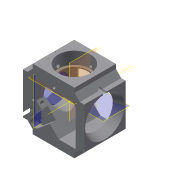
# Autodesk Inventor part: 20_Cube_Insert_Filter_25mm
Saved by Autodesk Inventor 2022 (Build 260153000, 153)
## iProperties
Created: 2019-07-01
Part Number: 20_Cube_Insert_Filter_25mm
Material: Generic
Document SubType Name: Modeling
Designer: diederichbenedict
Density: 1 g/cm^3
Appearance: Default
Author: diederichbenedict
Autodesk Inventor part; units mm, degrees
ref_plane "YZ Plane" through (0, 0, 0) normal (1, 0, 0) x (0, 1, 0)
ref_plane "Work Plane1" through (0, 0, 10) normal (0, 0, 1) x (1, 0, 0)
sketch "Sketch1" plane through (0, 0, 10) normal (0, 0, 1) x (1, 0, 0)
  line L0 (-4.029928, -0.353838) -> (-2.232156, 1.443934) construction
  arc A0 (-1.443934, 2.232156) -> (-2.232156, 1.443934) centre (-0.929928, 0.929928) ccw construction
  line L1 (-1.443934, 2.232156) -> (0.353838, 4.029928) construction
  line L2 (-37.829928, 42.829928) -> (-37.829928, 37.829928) construction
  line L3 (-37.829928, 37.829928) -> (-42.920801, 37.829928) construction
  line L4 (-37.829928, 42.213694) -> (-37.829928, 45.829928) construction
  line L5 (-37.829928, 45.829928) -> (-4.029928, 45.829928) construction
  line L6 (-4.029928, 45.829928) -> (-4.029928, 42.213694) construction
  line L7 (-4.029928, 4.029928) -> (0.353838, 4.029928)
  circle A1 centre (-20.929928, 20.929928) radius 17.5
  line L8 (-20.929928, 58.972273) -> (17.112417, 20.929928) construction
  line L9 (17.112417, 20.929928) -> (-20.929928, -17.112417) construction
  line L10 (-20.929928, -17.112417) -> (-58.972273, 20.929928) construction
  line L11 (-58.972273, 20.929928) -> (-20.929928, 58.972273) construction
  line L12 (-20.929928, 58.972273) -> (-20.929928, -17.112417) construction
  line L13 (17.112417, 20.929928) -> (-58.972273, 20.929928) construction
  line L14 (-20.929928, 58.972273) -> (32.870072, 58.972273) construction
  line L15 (-43.429928, 43.429928) -> (1.570072, 43.429928) construction
  line L16 (1.570072, 43.429928) -> (1.570072, -1.570072) construction
  line L17 (1.570072, -1.570072) -> (-43.429928, -1.570072) construction
  line L18 (-43.429928, -1.570072) -> (-43.429928, 43.429928) construction
  line L19 (-43.429928, 43.429928) -> (1.570072, -1.570072) construction
  line L20 (1.570072, 43.429928) -> (-43.429928, -1.570072) construction
  line L21 (-43.429928, 5.387583) -> (-43.429928, 36.472273)
  line L22 (-43.429928, 36.472273) -> (-36.472273, 43.429928)
  line L23 (-36.472273, 43.429928) -> (-5.387583, 43.429928)
  line L24 (-5.387583, 43.429928) -> (1.570072, 36.472273)
  line L25 (1.570072, 36.472273) -> (1.570072, 5.387583)
  line L26 (1.570072, 5.387583) -> (-5.387583, -1.570072)
  line L27 (-5.387583, -1.570072) -> (-36.472273, -1.570072)
  line L28 (-36.472273, -1.570072) -> (-43.429928, 5.387583)
  line L29 (-4.029928, 42.213694) -> (-37.829928, 42.213694)
  line L30 (-4.029928, -0.353838) -> (-4.029928, 4.029928)
  circle A2 centre (-20.929928, 20.929928) radius 1.5
  line L31 (-10.929928, 10.929928) -> (-30.929928, 10.929928) construction
  line L32 (-30.929928, 10.929928) -> (-30.929928, 30.929928) construction
  line L33 (-30.929928, 30.929928) -> (-10.929928, 30.929928) construction
  line L34 (-10.929928, 30.929928) -> (-10.929928, 10.929928) construction
  line L35 (-10.929928, 10.929928) -> (-30.929928, 30.929928) construction
  line L36 (-30.929928, 10.929928) -> (-10.929928, 30.929928) construction
  circle A3 centre (-30.929928, 30.929928) radius 1.4
  circle A4 centre (-30.929928, 10.929928) radius 1.4
  circle A5 centre (-10.929928, 10.929928) radius 1.4
  line L37 (-45.829928, 37.829928) -> (-42.072273, 37.829928) construction
  line L38 (-42.172273, 37.729928) -> (-45.829928, 37.729928)
  line L39 (-45.829928, 37.729928) -> (-45.829928, 4.129928)
  line L40 (-45.829928, 4.129928) -> (-42.172273, 4.129928)
  line L41 (-42.172273, 4.129928) -> (-42.172273, 37.729928)
  line L42 (-45.829928, 4.029928) -> (-42.072273, 4.029928) construction
  line L43 (-45.829928, 37.829928) -> (-42.072273, 37.829928)
  line L44 (-37.729928, 45.829928) -> (-4.129928, 45.829928)
  line L45 (-4.129928, 45.829928) -> (-4.129928, 42.172273)
  line L46 (-4.129928, 42.172273) -> (-37.729928, 42.172273)
  line L47 (-37.729928, 42.172273) -> (-37.729928, 45.829928)
  line L48 (0.470072, 37.829928) -> (0.470072, 4.029928) construction
  line L49 (0.470072, 4.029928) -> (3.970072, 4.029928) construction
  line L50 (3.970072, 37.829928) -> (3.970072, 4.029928) construction
  line L51 (0.470072, 37.829928) -> (3.970072, 37.829928) construction
  line L52 (-45.829928, -3.970072) -> (-4.029928, -3.970072) construction
  line L53 (0.312417, 37.729928) -> (3.970072, 37.729928)
  line L54 (3.970072, 37.729928) -> (3.970072, 4.129928)
  line L55 (3.970072, 4.129928) -> (0.312417, 4.129928)
  line L56 (0.312417, 4.129928) -> (0.312417, 37.729928)
  line L57 (-4.171349, -0.353838) -> (-37.729928, -0.353838)
  line L58 (-37.729928, -0.353838) -> (-37.729928, -3.970072)
  line L59 (-37.729928, -3.970072) -> (-4.171349, -3.970072)
  line L60 (-4.171349, -3.970072) -> (-4.171349, -0.353838)
  point P0 (-37.829928, 4.029928)
  dimension "d18" = 53.8
  dimension "d19" = 45
  dimension "d20" = 53.8
  dimension "d21" = 45
  dimension "d22" = 45
  dimension "d30" = 20
  dimension "d31" = 20
  dimension "d32" = 2.8
  dimension "d33" = 2.8
  dimension "d34" = 2.8
  dimension "d35" = 3
  dimension "d36" = 0.1
  dimension "d37" = 0.1
  dimension "d38" = 0.1
  dimension "d39" = 0.1
  constraints: 86 end point, 21 point on line, 14 parallel, 8 perpendicular, 7 horizontal, 7 midpoint, 4 centre point, 4 coincident, 1 equal length
  measures "d18" distance of L8.start L8.end
  measures "d19" angle of L8 L14
  measures "d20" distance of L8.end L9.end
  measures "d21" distance of L16.end L17.end
  measures "d22" distance of L15.end L16.end
  measures "d30" distance of L32.end L33.end
  measures "d31" distance of L31.end L32.end
  measures "d32" diameter of A3
  measures "d33" diameter of A4
  measures "d34" diameter of A5
  measures "d35" diameter of A2
  measures "d36" distance between parallel lines of L38 L43
  measures "d37" distance between parallel lines of L40 L42
  measures "d38" distance between parallel lines of L45 L6
  measures "d39" distance between parallel lines of L4 L47
sketch "Sketch1 outline for Extrusion1" plane through (0, 0, 10) normal (0, 0, 1) x (1, 0, 0)
  line L0 (-37.729928, -3.970072) -> (-4.171349, -3.970072)
  line L1 (-4.171349, -3.970072) -> (-4.171349, -0.353838)
  line L2 (0.312417, 4.129928) -> (-4.171349, -0.353838)
  line L3 (0.312417, 4.129928) -> (3.970072, 4.129928)
  line L4 (3.970072, 4.129928) -> (3.970072, 37.729928)
  line L5 (3.970072, 37.729928) -> (0.312417, 37.729928)
  line L6 (-4.129928, 42.172273) -> (0.312417, 37.729928)
  line L7 (-4.129928, 42.172273) -> (-4.129928, 45.829928)
  line L8 (-4.129928, 45.829928) -> (-37.729928, 45.829928)
  line L9 (-37.729928, 45.829928) -> (-37.729928, 42.172273)
  line L10 (-42.172273, 37.729928) -> (-37.729928, 42.172273)
  line L11 (-42.172273, 37.729928) -> (-45.829928, 37.729928)
  line L12 (-45.829928, 37.729928) -> (-45.829928, 4.129928)
  line L13 (-45.829928, 4.129928) -> (-42.172273, 4.129928)
  line L14 (-37.688507, -0.353838) -> (-42.172273, 4.129928)
  line L15 (-37.688507, -0.353838) -> (-37.729928, -0.353838)
  line L16 (-37.729928, -0.353838) -> (-37.729928, -3.970072)
extrude "Extrusion1" add sketch "Sketch1 outline for Extrusion1" along normal blind 33.8
sketch "Skizze4" plane through (0, 0, 43.8) normal (0, 0, 1) x (1, 0, 0)
  line L0 (-37.729928, 42.172273) -> (-42.172273, 37.729928)
  line L1 (-42.172273, 37.729928) -> (-45.829928, 37.729928)
  line L2 (-45.829928, 37.729928) -> (-45.829928, 4.129928) construction
  line L3 (-45.829928, 4.129928) -> (-42.172273, 4.129928)
  line L4 (-42.172273, 4.129928) -> (-37.688507, -0.353838)
  line L5 (-37.688507, -0.353838) -> (-37.729928, -0.353838)
  line L6 (-37.729928, -0.353838) -> (-37.729928, -3.970072)
  line L7 (-37.729928, -3.970072) -> (-4.171349, -3.970072) construction
  line L8 (-4.171349, -3.970072) -> (-4.171349, -0.353838)
  line L9 (-4.171349, -0.353838) -> (0.312417, 4.129928)
  line L10 (0.312417, 4.129928) -> (3.970072, 4.129928)
  line L11 (3.970072, 4.129928) -> (3.970072, 37.729928) construction
  line L12 (3.970072, 37.729928) -> (0.312417, 37.729928)
  line L13 (0.312417, 37.729928) -> (-4.129928, 42.172273)
  line L14 (-4.129928, 42.172273) -> (-4.129928, 45.829928)
  line L15 (-4.129928, 45.829928) -> (-37.729928, 45.829928) construction
  line L16 (-37.729928, 45.829928) -> (-37.729928, 42.172273)
  line L17 (-37.929928, 46.029928) -> (-3.929928, 46.029928) construction
  line L18 (-3.929928, 46.029928) -> (-3.929928, 42.255116)
  line L19 (-3.929928, 42.255116) -> (0.39526, 37.929928)
  line L20 (0.39526, 37.929928) -> (4.170072, 37.929928)
  line L21 (4.170072, 37.929928) -> (4.170072, 3.929928) construction
  line L22 (4.170072, 3.929928) -> (0.39526, 3.929928)
  line L23 (0.39526, 3.929928) -> (-3.971349, -0.436681)
  line L24 (-3.971349, -0.436681) -> (-3.971349, -4.170072)
  line L25 (-3.971349, -4.170072) -> (-37.929928, -4.170072) construction
  line L26 (-37.929928, -4.170072) -> (-37.929928, -0.39526)
  line L27 (-37.929928, -0.39526) -> (-42.255116, 3.929928)
  line L28 (-42.255116, 3.929928) -> (-46.029928, 3.929928)
  line L29 (-46.029928, 3.929928) -> (-46.029928, 37.929928) construction
  line L30 (-46.029928, 37.929928) -> (-42.255116, 37.929928)
  line L31 (-42.255116, 37.929928) -> (-37.929928, 42.255116)
  line L32 (-37.929928, 42.255116) -> (-37.929928, 46.029928)
  line L33 (-45.829928, 37.729928) -> (-45.829928, 37.929928)
  line L34 (-4.129928, 45.829928) -> (-37.729928, 45.829928)
  line L35 (-37.729928, 45.829928) -> (-37.929928, 45.829928)
  line L36 (-4.129928, 45.829928) -> (-3.929928, 45.829928)
  line L37 (3.970072, 37.729928) -> (3.970072, 37.929928)
  line L38 (3.970072, 4.129928) -> (3.970072, 37.729928)
  line L39 (3.970072, 4.129928) -> (3.970072, 3.929928)
  line L40 (-4.171349, -3.970072) -> (-3.971349, -3.970072)
  line L41 (-37.729928, -3.970072) -> (-37.929928, -3.970072)
  line L42 (-45.829928, 4.129928) -> (-45.829928, 3.929928)
  point P0 (0, 0)
  dimension "d40" = 0.2
  constraints: 48 end point, 12 point on line, 4 perpendicular, 15 other
  measures "d40" distance between parallel lines of L15 L17
extrude "IM_offset" add sketch "Skizze4" against normal up to surface (33.8 mm away)
ref_plane "Arbeitsebene12" through (-37.929928, 20.929928, 10) normal (0, -1, 0) x (1, 0, 0)
ref_plane "Arbeitsebene13" through (-20.929928, 3.929928, 10) normal (1, 0, 0) x (0, 0, -1)
sketch "Skizze39" plane through (-37.929928, 45.829928, 10) normal (0, 1, 0) x (1, 0, 0)
  circle A0 centre (17.08, -16.97) radius 13.3985 construction
  circle A1 centre (17.08, -16.97) radius 13.15
  point P0 (37.929928, 10)
  dimension "d259" = 26.3
  constraints: 1 centre point, 1 coincident
  measures "d259" diameter of A1
ref_plane "Arbeitsebene14" through (-33.740428, 34.239928, 14.0795) normal (0, -1, 0) x (1, 0, 0)
extrude "Extrusion34" cut sketch "Skizze39" against normal blind 11.1
sketch "Skizze40" plane through (-45.829928, 3.929928, 10) normal (-1, 0, 0) x (0, 0, 1)
  circle A0 centre (16.97, 17) radius 13.1445 construction
  circle A1 centre (16.97, 17) radius 13.15
  point P0 (-10, -3.929928)
  dimension "d258" = 26.3
  constraints: 1 centre point, 1 coincident
  measures "d258" diameter of A1
extrude "Extrusion35" cut sketch "Skizze40" against normal blind 11.1
sketch "Skizze41" plane through (3.970072, 3.929928, 10) normal (1, 0, 0) x (0, 0, -1)
  line L0 (0, 34) -> (0, 0) projected
  line L1 (-33.8, 34) -> (0, 34) projected
  line L2 (-33.8, 0) -> (-33.8, 34) projected
  line L3 (-33.8, 0) -> (0, 0) projected
  circle A0 centre (-16.97, 17) radius 12.8905 projected
  circle A1 centre (-16.97, 17) radius 10
  point P0 (10, -3.929928)
  dimension "d201" = 20
  constraints: 1 centre point, 1 coincident
  measures "d201" diameter of A1
extrude "Extrusion36" cut sketch "Skizze41" against normal through all contours A1
sketch "Skizze42" plane through (-20.849928, 34.729928, 26.97) normal (0, 1, 0) x (1, 0, 0)
  circle A0 centre (0, 0) radius 13.3985 projected
  circle A1 centre (0, 0) radius 10
  point P0 (20.849928, 26.97)
  dimension "d204" = 20
  constraints: 1 centre point, 1 coincident
  measures "d204" diameter of A1
extrude "Extrusion37" cut sketch "Skizze42" against normal blind 14 contours A1
sketch "Skizze45" plane through (0, 0, 43.8) normal (0, 0, 1) x (1, 0, 0)
  line L0 (-3.029928, 3.029928) -> (-35.029928, 3.029928)
  line L1 (-35.029928, 3.029928) -> (-35.029928, 35.029928)
  line L2 (-35.029928, 35.029928) -> (-5.585351, 35.029928)
  line L3 (-3.029928, 35.029928) -> (-3.029928, 3.029928)
  line L4 (-3.029928, 3.029928) -> (-35.029928, 35.029928) construction
  line L5 (-35.029928, 3.029928) -> (-3.029928, 35.029928) construction
  line L6 (-3.971349, -3.970072) -> (-37.929928, -3.970072)
  line L7 (3.970072, 3.929928) -> (3.970072, 37.929928)
  line L8 (-5.585351, 35.029928) -> (-3.029928, 32.474505)
  line L9 (-37.929928, -0.39526) -> (-42.255116, 3.929928)
  line L10 (-35.029928, 21.414704) -> (-16.645152, 3.029928)
  point P0 (-20.649928, 20.729928)
  point P1 (-19.029928, 19.029928)
  dimension "d241" = 32
  dimension "d242" = 32
  dimension "d243" = 7
  dimension "d244" = 7
  dimension "d283" = 1.80696
  dimension "d284" = 45
  dimension "d285" = 13
  constraints: 16 end point, 3 parallel, 3 point on line, 2 midpoint, 1 horizontal, 1 perpendicular
  measures "d241" distance of L1.end L3.start
  measures "d242" distance of L0.end L1.end
  measures "d243" distance between parallel lines of L0 L6
  measures "d244" distance between parallel lines of L7 L3
  measures "d283" distance from line of L3.start L8
  measures "d284" angle of L0 L10
  measures "d285" distance from line of L0.end L10
extrude "Extrusion38" cut sketch "Skizze45" against normal through all contours L0 L10 L1 L2 L8 L3
sketch "Skizze46" plane through (3.970072, 3.929928, 10) normal (1, 0, 0) x (0, 0, -1)
  circle A0 centre (-16.97, 17) radius 10
  circle A1 centre (-16.97, 17) radius 13.1445
  circle A2 centre (-16.97, 17) radius 16.057916
  point P0 (10, -3.929928)
  point P1 (-25.571304, 7.06041)
  point P2 (-8.368696, 7.06041)
  constraints: 1 centre point, 1 coincident
sketch "Skizze46 outline for Extrusion39" plane through (3.970072, 3.929928, 10) normal (1, 0, 0) x (0, 0, -1)
  circle A0 centre (-16.97, 17) radius 16.057916
extrude "Extrusion39" cut sketch "Skizze46 outline for Extrusion39" against normal blind 16 draft -20
ref_plane "Arbeitsebene15" through (-35.829928, 3.929928, 10) normal (-1, 0, 0) x (0, 0, 1)
ref_plane "Arbeitsebene16" through (-37.929928, 35.829928, 10) normal (0, 1, 0) x (1, 0, 0)
sketch "Skizze49" plane through (-37.929928, 35.829928, 10) normal (0, 1, 0) x (1, 0, 0)
  line L0 (41.9, -0.912084) -> (41.9, -33.027916)
  circle A0 centre (17.08, -16.97) radius 13.15
  circle A1 centre (17.08, -16.97) radius 11
  point P0 (37.929928, 10)
  dimension "d262" = 22
  constraints: 1 centre point, 1 coincident
  measures "d262" diameter of A1
extrude "Extrusion41" add sketch "Skizze49" against normal up to surface (0.8 mm away)
ref_plane "Arbeitsebene17" through (-35.829928, 3.929928, 10) normal (-1, 0, 0) x (0, 0, 1)
sketch "Skizze51" plane through (-35.829928, 3.929928, 10) normal (-1, 0, 0) x (0, 0, 1)
  circle A0 centre (16.97, 17) radius 13.15 projected
  circle A1 centre (16.97, 17) radius 11
  point P0 (-10, -3.929928)
  dimension "d266" = 22
  constraints: 1 centre point, 1 coincident
  measures "d266" diameter of A1
extrude "Extrusion42" add sketch "Skizze51" against normal up to surface (0.8 mm away)
sketch "Skizze52" plane through (-45.829928, 3.929928, 43.8) normal (0, -1, 0) x (1, 0, 0)
  line L0 (10, -29.98) -> (10, -3.68)
  line L1 (0, -29.98) -> (0, -3.68)
  circle A0 centre (24.98, -16.83) radius 11
  circle A1 centre (8.042431, -16.83) radius 1.45
  point P0 (45.829928, -43.8)
  dimension "d269" = 2.9
  constraints: 1 centre point
  measures "d269" diameter of A1
extrude "Extrusion43" cut sketch "Skizze52" along normal mid plane 20 contours A1
pattern_circular "Runde Anordnung2" count 4 over 360 about axis through (-45.829928, 20.929928, 26.97) along (1, 0, 0) of "Extrusion43"
pattern_circular "Runde Anordnung3" count 2 over 90 about axis through (-20.929928, 20.929928, 10) along (0, 0, -1) of "Extrusion43", "Runde Anordnung2"
sketch "Skizze48" plane through (-36.142522, -2.182666, 10) normal (-0.7071068, -0.7071068, 0) x (0.7071068, -0.7071068, 0)
  ellipse E0 centre (0.100714, 16.97) end of major axis (0.100714, 15.52) minor radius 1.025305 (0, 15.527012) -> (0, 18.412988) ccw
  line L0 (0, 15.527012) -> (0, 0)
  line L1 (24.012341, 0) -> (0, 0)
  line L2 (24.012341, 33.8) -> (24.012341, 0)
  line L3 (24.012341, 33.8) -> (0, 33.8)
  line L4 (0, 33.8) -> (0, 18.412988)
  ellipse E1 centre (-2.326346, 16.97) end of major axis (-0.275736, 16.97) minor radius 1.45 (-2.527774, 18.412988) -> (-2.527774, 15.527012) ccw
  line L5 (-2.527774, 33.8) -> (-2.527774, 18.412988)
  line L6 (-2.527774, 33.8) -> (-8.644513, 33.8)
  line L7 (-8.644513, 33.8) -> (-8.644513, 0)
  line L8 (-2.527774, 0) -> (-8.644513, 0)
  line L9 (-2.527774, 15.527012) -> (-2.527774, 0)
  circle A0 centre (-12.899286, 30.97) radius 2.245162
  circle A1 centre (8.100714, 16.97) radius 3.838969
  line L10 (0, 15.527012) -> (0, 0)
  point P0 (24.013244, -10)
  point P1 (-12.899286, 2.97)
  dimension "d286" = 14
  dimension "d287" = 14
  dimension "d288" = 0
  dimension "d289" = 13
  dimension "d290" = 8
  dimension "d291" = 0
  constraints: 2 centre point, 2 coincident, 2 other
  measures "d286" vertical distance of point (8.101, 16.97) point (-12.899, 30.97)
  measures "d287" vertical distance of point (-12.899, 2.97) point (8.101, 16.97)
  measures "d288" vertical distance of point (8.101, 16.97) point (0.101, 16.97)
  measures "d289" horizontal distance of point (0.101, 16.97) point (-12.899, 30.97)
  measures "d290" distance of point (0.101, 16.97) point (8.101, 16.97)
  measures "d291" horizontal distance of point (-12.899, 2.97) A0.centre
hole "Bohrung3" at (-45.263694, 6.938507, 40.97) at (-45.263694, 6.938507, 12.97) at (-30.414452, -7.910736, 26.97) direction (0.7071068, 0.7071068, 0) diameter 2.8 depth 20 tip angle 118 counterbore diameter 6 counterbore depth 10
sketch "Skizze54" plane through (-42.255116, 3.929928, 43.8) normal (-0.7071068, -0.7071068, 0) x (-0.7071068, 0.7071068, 0)
  arc A0 (5.250313, 0) -> (5.055548, 5.721152) centre (4.254773, 2.83) ccw
  arc A1 (5.055548, 27.938848) -> (5.055548, 33.721152) centre (4.254773, 30.83) ccw
  circle A2 centre (4.254773, 2.83) radius 3
  circle A3 centre (4.254773, 30.83) radius 3
  point P0 (-32.657758, 43.8)
  point P1 (5.055548, 0.438848)
  point P2 (5.055548, 33.721152)
  point P3 (5.055548, 27.938848)
  point P4 (5.055548, 5.721152)
  point P5 (7.254773, 2.83)
  point P6 (5.250313, 0)
  constraints: 2 centre point, 2 coincident, 2 concentric
extrude "Extrusion45" cut sketch "Skizze54" along normal blind 10
sketch "Skizze55" plane through (0, 0, 43.8) normal (0, 0, 1) x (1, 0, 0)
  line L0 (-16.645152, 3.029928) -> (-35.029928, 21.414704)
  line L1 (-35.029928, 21.414704) -> (-35.029928, 35.029928)
  line L2 (-35.029928, 35.029928) -> (-5.585351, 35.029928)
  line L3 (-5.585351, 35.029928) -> (-3.029928, 32.474505)
  line L4 (-3.029928, 32.474505) -> (-3.029928, 3.029928)
  line L5 (-3.029928, 3.029928) -> (-16.645152, 3.029928)
  circle A0 centre (-37.787497, 20.929928) radius 1.45
  circle A1 centre (-20.929928, 37.787497) radius 1.45
  line L6 (-37.488673, 13.305621) -> (-45.829928, 4.964367)
  line L7 (-45.829928, 4.964367) -> (-45.829928, 3.929928)
  line L8 (-42.255116, 3.929928) -> (-45.829928, 3.929928)
  line L9 (-37.929928, -0.39526) -> (-42.255116, 3.929928)
  line L10 (-37.929928, -3.970072) -> (-37.929928, -0.39526)
  line L11 (-3.971349, -3.970072) -> (-37.929928, -3.970072)
  line L12 (-3.971349, -3.970072) -> (-3.971349, -0.436681)
  line L13 (-3.971349, -0.436681) -> (0.39526, 3.929928)
  line L14 (0.39526, 3.929928) -> (3.970072, 3.929928)
  line L15 (3.970072, 3.929928) -> (3.970072, 37.929928)
  line L16 (3.970072, 37.929928) -> (0.39526, 37.929928)
  line L17 (0.39526, 37.929928) -> (-3.929928, 42.255116)
  line L18 (-3.929928, 42.255116) -> (-3.929928, 45.829928)
  line L19 (-3.929928, 45.829928) -> (-37.929928, 45.829928)
  line L20 (-37.929928, 45.829928) -> (-37.929928, 42.255116)
  line L21 (-37.929928, 42.255116) -> (-42.255116, 37.929928)
  line L22 (-42.255116, 37.929928) -> (-45.829928, 37.929928)
  line L23 (-45.829928, 37.929928) -> (-45.829928, 7.780179)
  line L24 (-45.829928, 7.780179) -> (-38.89658, 14.713528)
  line L25 (-38.89658, 14.713528) -> (-37.488673, 13.305621)
  circle A2 centre (-22.580635, 15.823687) radius 1.45
  circle A3 centre (-36.172868, 5.056468) radius 1.4
  line L26 (-3.929928, 42.255116) -> (0.39526, 37.929928)
  line L27 (-1.452074, 39.777262) -> (-39.777262, 1.452074)
  point P0 (0, 0)
  dimension "d294" = 2.8
  constraints: 3 point on line, 2 end point, 1 centre point, 1 perpendicular
  measures "d294" diameter of A3
extrude "Extrusion46" cut sketch "Skizze55" against normal through all contours L27 A3 | A3 L27
sketch "Skizze56" plane through (0, 0, 43.8) normal (0, 0, 1) x (1, 0, 0)
  circle A0 centre (-36.172868, 5.056468) radius 1.4
  circle A1 centre (-36.172868, 5.056468) radius 3.719273
  line L0 (-35.029928, 21.414704) -> (-16.645152, 3.029928)
  line L1 (-18.987387, 5.372164) -> (-32.136053, 18.520829)
  line L2 (-3.971349, -3.970072) -> (-37.929928, -3.970072)
  line L3 (-33.782165, 2.207339) -> (-24.016733, 10.40151)
  line L4 (-39.021996, 7.44717) -> (-30.827826, 17.212602)
  line L5 (-45.829928, 37.929928) -> (-45.829928, 7.780179)
  line L6 (-37.929928, -0.39526) -> (-42.255116, 3.929928)
  line L7 (-40.092522, 1.767334) -> (-4.30764, 33.752217) construction
  line L8 (-3.029928, 32.474505) -> (-5.585351, 35.029928)
  point P0 (0, 0)
  point P1 (-34.252225, 1.871484)
  point P2 (-39.671903, 6.31732)
  point P3 (-30.827826, 17.212602)
  dimension "d299" = 40
  dimension "d300" = 140
  constraints: 8 end point, 4 point on circle, 4 point on line, 2 midpoint, 2 tangent, 1 centre point, 1 collinear
  measures "d299" angle of L2 L3
  measures "d300" angle of L5 L4
extrude "Extrusion47" cut sketch "Skizze56" against normal blind 5
sketch "Skizze57" plane through (0, 0, 10) normal (0, 0, -1) x (-1, 0, 0)
  arc A0 (33.782165, 2.207339) -> (39.021996, 7.44717) centre (36.172868, 5.056468) ccw
  line L0 (24.016733, 10.40151) -> (33.782165, 2.207339)
  line L1 (30.827826, 17.212602) -> (24.016733, 10.40151)
  line L2 (39.021996, 7.44717) -> (30.827826, 17.212602)
  circle A1 centre (36.172868, 5.056468) radius 1.4
  point P0 (0, 0)
extrude "Extrusion48" cut sketch "Skizze57" against normal blind 5
body "Solid1"
